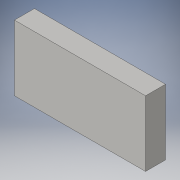
# Autodesk Inventor part: BackSupport
Saved by Autodesk Inventor 2016 (Build 200138000, 138)
## iProperties
Created: 2015-11-25
Part Number: BackSupport
Material: Generic
Document SubType Name: Modeling
Designer: sfeng
Density: 1 g/cm^3
Appearance: Default
Author: sfeng
Autodesk Inventor part; units mm, degrees
ref_plane "YZ Plane" through (0, 0, 0) normal (1, 0, 0) x (0, 1, 0)
ref_plane "XZ Plane" through (0, 0, 0) normal (0, 1, 0) x (-1, 0, 0)
ref_plane "XY Plane" through (0, 0, 0) normal (0, 0, 1) x (1, 0, 0)
sketch "Sketch1" plane through (0, 0, 0) normal (0, 0, 1) x (1, 0, 0)
  line L0 (-1002.627, 279.3345) -> (497.373, 279.3345)
  line L1 (497.373, 279.3345) -> (497.373, -470.6655)
  line L2 (497.373, -470.6655) -> (-1002.627, -470.6655)
  line L3 (-1002.627, -470.6655) -> (-1002.627, 279.3345)
  point P0 (0, 0)
  dimension "d0" = 1500
  dimension "d1" = 750
  constraints: 8 end point, 2 parallel, 1 horizontal, 1 perpendicular
  measures "d0" distance of L0.start L0.end
  measures "d1" distance of L0.end L1.end
extrude "Extrusion1" add sketch "Sketch1" along normal blind 228.6
body "Solid1"
